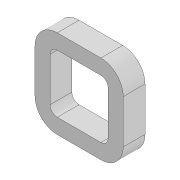
# Autodesk Inventor part: Peça49
Saved by Autodesk Inventor 2020 (Build 240168000, 168)
## iProperties
Created: 2022-07-18
Part Number: Peça49
Material: Genérico
Document SubType Name: Modeling
Designer: gabri
Density: 1 g/cm^3
Appearance: Padrão
Author: gabri
Autodesk Inventor part; units mm, degrees
ref_plane "YZ Plane" through (0, 0, 0) normal (1, 0, 0) x (0, 1, 0)
ref_plane "XZ Plane" through (0, 0, 0) normal (0, 1, 0) x (-1, 0, 0)
ref_plane "Plano de trabalho1" through (0, 0, 0) normal (0, 0, 1) x (1, 0, 0)
sketch "Esboço1" plane through (0, 0, 0) normal (0, 0, 1) x (1, 0, 0)
  arc A0 (-38.9725, -30.5146) -> (-28.9725, -40.5146) centre (-28.9725, -30.5146) ccw projected
  line L0 (31.0275, -40.5146) -> (-28.9725, -40.5146) projected
  arc A1 (31.0275, -40.5146) -> (41.0275, -30.5146) centre (31.0275, -30.5146) ccw projected
  line L1 (41.0275, 29.4854) -> (41.0275, -30.5146) projected
  arc A2 (41.0275, 29.4854) -> (31.0275, 39.4854) centre (31.0275, 29.4854) ccw projected
  line L2 (-28.9725, 39.4854) -> (31.0275, 39.4854) projected
  arc A3 (-28.9725, 39.4854) -> (-38.9725, 29.4854) centre (-28.9725, 29.4854) ccw projected
  line L3 (-38.9725, -30.5146) -> (-38.9725, 29.4854) projected
  circle A4 centre (1.0275, -0.5146) radius 5 projected
  arc A5 (-52.2205, -30.5146) -> (-28.9725, -53.7625) centre (-28.9725, -30.5146) ccw
  line L4 (-52.2205, -30.5146) -> (-52.2205, 29.4854)
  arc A6 (-28.9725, 52.7334) -> (-52.2205, 29.4854) centre (-28.9725, 29.4854) ccw
  line L5 (-28.9725, 52.7334) -> (31.0275, 52.7334)
  arc A7 (54.2754, 29.4855) -> (31.0275, 52.7334) centre (31.0275, 29.4854) ccw
  line L6 (54.2754, 29.4855) -> (54.2754, -30.5145)
  arc A8 (31.0275, -53.7625) -> (54.2754, -30.5145) centre (31.0275, -30.5146) ccw
  line L7 (31.0275, -53.7625) -> (-28.9725, -53.7625)
  arc A9 (-59.6663, -30.5146) -> (-28.9725, -61.2084) centre (-28.9725, -30.5146) ccw
  line L8 (-59.6663, -30.5146) -> (-59.6664, 29.4854)
  arc A10 (-28.9725, 60.1793) -> (-59.6664, 29.4854) centre (-28.9725, 29.4854) ccw
  line L9 (-28.9725, 60.1793) -> (31.0275, 60.1793)
  arc A11 (61.7213, 29.4855) -> (31.0275, 60.1793) centre (31.0275, 29.4854) ccw
  line L10 (61.7213, 29.4855) -> (61.7213, -30.5145)
  arc A12 (31.0275, -61.2084) -> (61.7213, -30.5145) centre (31.0275, -30.5146) ccw
  line L11 (31.0275, -61.2084) -> (-28.9725, -61.2084)
  point P0 (0, 0)
  constraints: 16 end point, 16 point on circle, 8 centre point, 14 other
extrude "Extrusão1" add sketch "Esboço1" along normal blind 30 contours L4 A6 L5 A7 L6 A8 L7 A5 | L8 A10 L9 A11 L10 A12 L11 A9
